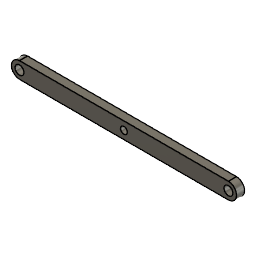
barra_direccion_v3 (Autodesk Fusion 360 design; units mm, degrees)
part number: 2026-03-15-19-52-01-353
Autodesk Fusion 360 part; units mm, degrees
sketch "Boceto1" plane through (0, 0, 0) normal (0, 0, 1) x (1, 0, 0)
  line L0 (0, -23.8223) -> (0, 23.8223) construction
  circle A0 centre (64.256, 0) radius 2.75
  circle A1 centre (-64.256, 0) radius 2.75
  line L1 (-64.256, 5) -> (64.256, 5)
  line L2 (0, 0) -> (11, 0) construction
  line L3 (-64.256, -5) -> (64.256, -5)
  arc A2 (-64.256, 5) -> (-64.256, -5) centre (-64.256, 0) ccw
  arc A3 (64.256, -5) -> (64.256, 5) centre (64.256, 0) ccw
  dimension "d1" = 5.5
  dimension "d2" = 64.256
  dimension "d3" = 10
  dimension "d4" = 10
  dimension "d5" = 128.512
  constraint midpoint L0 L2.start
  constraint coincident L2.start origin
  constraint vertical L0
  constraint symmetric L0 A0 A1
  constraint concentric A1 A2
  constraint concentric A0 A3
  constraint tangent L1 A3
  constraint horizontal L1
  constraint perpendicular L0 L2
  constraint symmetric L1.start L2 L3.start
  constraint symmetric L1.end L2 L3.end
  measures "d1" diameter of A0
  measures "d2" distance of L2.start A0.centre
  measures "d3" diameter of A2
  measures "d4" diameter of A3
  measures "d5" distance of A1.centre A0.centre
extrude "Extruir1" add sketch "Boceto1" along normal blind 5
sketch "Boceto2" plane through (0, 0, 5) normal (0, 0, 1) x (1, 0, 0)
  circle A0 centre (64.256, 0) radius 2.75
  circle A1 centre (-64.256, 0) radius 2.75
  arc A2 (-64.256, 5) -> (-64.256, -5) centre (-64.256, 0) ccw
  line L0 (-64.256, -5) -> (64.256, -5)
  arc A3 (64.256, -5) -> (64.256, 5) centre (64.256, 0) ccw
  line L1 (64.256, 5) -> (-64.256, 5)
  circle A4 centre (0, 0) radius 2.1
  dimension "d8" = 4.2
  constraint coincident A4.centre origin
  measures "d8" diameter of A4
extrude "Extruir2" cut sketch "Boceto2" against normal through all contours A4
equation "d2 = ( 128.512 / 2 ) * 1 mm"
